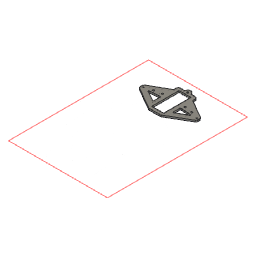
carBodyServoPlate v2 (Autodesk Fusion 360 design; units mm, degrees)
Autodesk Fusion 360 part; units mm, degrees
sketch "Sketch1" plane through (0, 0, 0) normal (0, 0, 1) x (1, 0, 0)
  line L0 (-11.5001, -26.5) -> (11.4999, -26.5)
  line L1 (11.4999, -26.5) -> (11.4999, 26.5)
  line L2 (11.4999, 26.5) -> (-11.5001, 26.5)
  line L3 (-11.5001, 26.5) -> (-11.5001, -26.5)
  line L4 (-0.0001, 26.5) -> (-0.0001, 31.5)
  circle A0 centre (-0.0001, 31.5) radius 1.6
  circle A1 centre (-0.0001, 31.5) radius 6
  line L5 (37.0364, 2.2639) -> (-37.0366, 2.2639)
  circle A2 centre (37.0364, 2.2639) radius 1.6
  circle A3 centre (-37.0366, 2.2639) radius 1.6
  circle A4 centre (-37.0366, 2.2639) radius 5
  circle A5 centre (37.0364, 2.2639) radius 5
  line L6 (-0.0001, 31.5) -> (37.0364, 2.2639)
  line L7 (-0.0001, 31.5) -> (-37.0366, 2.2639)
  line L8 (56, 1.4) -> (56, -6.6)
  line L9 (-56, -6.6) -> (-56, 1.4)
  line L10 (-18.5, 31.9382) -> (18.5, 31.9382)
  line L11 (18.5, 31.9382) -> (18.5, 22.9382)
  line L12 (-18.5, 22.9382) -> (-18.5, 31.9382)
  line L13 (-56, 1.4) -> (-18.5, 22.9382)
  line L14 (18.5, 22.9382) -> (56, 1.4)
  line L15 (11.4999, -32.5) -> (-11.5001, -32.5)
  line L16 (-11.5001, -32.5) -> (-56, -6.6)
  line L17 (11.4999, -32.5) -> (56, -6.6)
  line L18 (56, -2.6) -> (52, -2.6)
  circle A6 centre (52, -2.6) radius 1.1
  line L19 (-56, -2.6) -> (-52, -2.6)
  circle A7 centre (-52, -2.6) radius 1.1
  circle A8 centre (-22.0001, 4.7639) radius 5
  line L20 (-22.0001, 4.7639) -> (-22.0001, 2.2639)
  line L21 (-0.0001, 2.2639) -> (-22.0001, 2.2639)
  line L22 (-22.0001, 2.2639) -> (-22.0001, 4.7639)
  line L23 (-22.0001, 4.7639) -> (-0.0001, 4.7639)
  line L24 (-0.0001, 4.7639) -> (-0.0001, 2.2639)
  line L25 (-0.0001, 4.7639) -> (21.9999, 4.7639)
  line L26 (21.9999, 4.7639) -> (21.9999, 2.2639)
  line L27 (21.9999, 2.2639) -> (-0.0001, 2.2639)
  line L28 (-0.0001, 2.2639) -> (-0.0001, 4.7639)
  circle A9 centre (21.9999, 4.7639) radius 5
  circle A10 centre (-22.0001, 4.7639) radius 1.6
  circle A11 centre (21.9999, 4.7639) radius 1.6
  circle A12 centre (20, -15) radius 1
  circle A13 centre (-20, -15) radius 1
  circle A14 centre (-40, -4) radius 1
  circle A15 centre (-20, -2.5) radius 1
  line L29 (-20.0748, -1.5028) -> (-40.0748, -3.0028)
  circle A16 centre (20, -2.5) radius 1
  circle A17 centre (40, -4) radius 1
  line L30 (40.0748, -3.0028) -> (20.0748, -1.5028)
  line L31 (19, -2.5) -> (19, -15)
  line L32 (20.4819, -15.8762) -> (40.4819, -4.8762)
  line L33 (-19, -2.5) -> (-19, -15)
  line L34 (-40.4819, -4.8762) -> (-20.4819, -15.8762)
  dimension "d1" = 23
  dimension "d2" = 53
  dimension "d3" = 5
  dimension "d4" = 3.2
  dimension "d5" = 12
  dimension "d20" = 3.2
  dimension "d21" = 3.2
  dimension "d22" = 10
  dimension "d23" = 10
  dimension "d24" = 112
  dimension "d25" = 8
  dimension "d26" = 37
  dimension "d27" = 9
  dimension "d30" = 2.2
  dimension "d31" = 4
  dimension "d32" = 4
  dimension "d33" = 2.2
  dimension "d34" = 10
  dimension "d36" = 22
  dimension "d37" = 2.5
  dimension "d38" = 22
  dimension "d39" = 2.5
  dimension "d40" = 10
  dimension "d41" = 3.2
  dimension "d42" = 3.2
  dimension "d43" = 2
  dimension "d44" = 2
  dimension "d50" = 2
  dimension "d51" = 2
  constraint horizontal L0
  constraint vertical L1
  constraint horizontal L2
  constraint vertical L3
  constraint midpoint L2 L4.start
  constraint perpendicular L2 L4
  constraint coincident L4.end A0.centre
  constraint coincident L5.start A2.centre
  constraint coincident L5.end A3.centre
  constraint concentric A3 A4
  constraint concentric A2 A5
  constraint vertical L8
  constraint vertical L9
  constraint horizontal L10
  constraint vertical L11
  constraint vertical L12
  constraint horizontal L15
  constraint midpoint L8 L18.start
  constraint perpendicular L8 L18
  constraint coincident L18.end A6.centre
  constraint midpoint L9 L19.start
  constraint perpendicular L9 L19
  constraint coincident L19.end A7.centre
  constraint coincident A8.centre L20.start
  constraint coincident L5 L20.end
  constraint perpendicular L5 L20
  constraint horizontal L21
  constraint vertical L22
  constraint horizontal L23
  constraint vertical L24
  constraint midpoint L5 L21.start
  constraint horizontal L25
  constraint vertical L26
  constraint horizontal L27
  constraint vertical L28
  constraint coincident L25.end L26.start
  constraint concentric A8 A10
  constraint coincident A15 L29.start
  constraint coincident A14 L29.end
  constraint tangent A14 L29
  constraint coincident A17 L30.start
  constraint coincident A16 L30.end
  constraint tangent A16 L30
  constraint tangent A17 L30
  constraint coincident A16 L31.start
  constraint coincident A12 L31.end
  constraint tangent A12 L31
  constraint coincident A12 L32.start
  constraint coincident A17 L32.end
  constraint tangent A17 L32
  constraint tangent A15 L29
  constraint coincident A15 L33.start
  constraint coincident A13 L33.end
  constraint tangent A13 L33
  constraint tangent A15 L33
  constraint coincident A14 L34.start
  constraint coincident A13 L34.end
  constraint tangent A13 L34
  constraint tangent A14 L34
  constraint tangent A12 L32
  constraint tangent A16 L31
  measures "d1" distance of L0.start L0.end
  measures "d2" distance of L0.start L2.end
  measures "d3" distance of L4.start L4.end
  measures "d4" diameter of A0
  measures "d5" diameter of A1
  measures "d20" diameter of A2
  measures "d21" diameter of A3
  measures "d22" diameter of A4
  measures "d23" diameter of A5
  measures "d24" distance of L9.end L8.start
  measures "d25" distance of L9.end L9.start
  measures "d26" distance of L10.start L10.end
  measures "d27" distance of L10.start L12.start
  measures "d30" diameter of A6
  measures "d31" distance of L18.start L18.end
  measures "d32" distance of L19.start L19.end
  measures "d33" diameter of A7
  measures "d34" diameter of A8
  measures "d36" distance of A8.centre L23.end
  measures "d37" distance of L21.start L23.end
  measures "d38" distance of L23.end L25.end
  measures "d39" distance of L23.end L21.start
  measures "d40" diameter of A9
  measures "d41" diameter of A10
  measures "d42" diameter of A11
  measures "d43" diameter of A12
  measures "d44" diameter of A13
  measures "d50" diameter of A15
  measures "d51" diameter of A16
extrude "Extrude1" add sketch "Sketch1" along normal blind 3 contours L0 L1 L2 L3 A1 L5 A4 A5 L6 L7 L8 L9 L10 L11 L12 L13 L14 L15 L16 L17 A8 L21 L27 A9 | L3 L5 A8 L21 L23 | L1 L5 L25 L27 A9 | L3 L5 A4 L7 A8 L23 | L5 A8 L21 | L5 A8 L20 L21 L22 L23 A10 | L1 L5 A5 L6 L25 A9 | L5 L25 L26 L27 A9 A11 | L5 L27 A9 | L5 A8 L20 L22 L23 A10 | L5 L25 L26 A9 A11 | L2 A1 L7 | L5 A3 A4 L7 | L5 A3 A4 L7 | L2 A1 L6 | L5 A2 A5 L6 | L5 A2 A5 L6 | L2 L4 A0 A1 L7 | A0 A1 L7 L10 | L2 L4 A0 A1 L6 | A0 A1 L6 L10 | A0 A1 L10 makes body 1
fillet "Fillet1" radius 4 8 edges at (-18.5, 31.9382, 1.5) (18.5, 31.9382, 1.5) (-56, -6.6, 1.5) (-56, 1.4, 1.5) (-11.5001, -32.5, 1.5) (11.4999, -32.5, 1.5) (56, -6.6, 1.5) (56, 1.4, 1.5) on bodies 1
copy_body "Body->Comp1" bodies 1 removing the originals makes body 2 in component "carBodyServoPlate"
component "carBodyServoPlate" placed x (1, 0, 0) y (0, 1, 0) z (0, 0, 1) at (0, 0, 0)
named bodies: "carBodyServoPlate"
